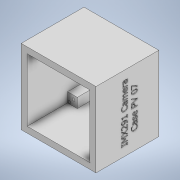
# Autodesk Inventor part: IMX291 Ethernet Strain Relief
Saved by Autodesk Inventor 2022.1 (Build 261234000, 234)
## iProperties
Created: 2021-07-23
Part Number: IMX291 Ethernet Strain Relief
Material: Generic
Document SubType Name: Modeling
Designer: robst
Density: 1 g/cm^3
Appearance: Default
Author: robst
Autodesk Inventor part; units mm, degrees
ref_plane "YZ Plane" through (0, 0, 0) normal (1, 0, 0) x (0, 1, 0)
ref_plane "XZ Plane" through (0, 0, 0) normal (0, 1, 0) x (-1, 0, 0)
ref_plane "XY Plane" through (0, 0, 0) normal (0, 0, 1) x (1, 0, 0)
sketch "Sketch8" plane through (0, 0, 0) normal (0, 0, 1) x (1, 0, 0)
  line L0 (-17, -17) -> (17, -17) construction
  line L1 (17, -17) -> (17, 17) construction
  line L2 (17, 17) -> (-17, 17) construction
  line L3 (-17, 17) -> (-17, -17) construction
  line L4 (-17, -17) -> (17, 17) construction
  line L5 (17, -17) -> (-17, 17) construction
  circle A0 centre (-17, 17) radius 0.889
  circle A1 centre (17, 17) radius 0.889
  circle A2 centre (17, -17) radius 0.889
  circle A3 centre (-17, -17) radius 0.889
  line L6 (-21, -21) -> (21, -21)
  line L7 (21, -21) -> (21, 21)
  line L8 (21, 21) -> (-21, 21)
  line L9 (-21, 21) -> (-21, -21)
  line L10 (-21, -21) -> (21, 21) construction
  line L11 (21, -21) -> (-21, 21) construction
  line L12 (-25, -25) -> (25, -25)
  line L13 (25, -25) -> (25, 25)
  line L14 (25, 25) -> (-25, 25)
  line L15 (-25, 25) -> (-25, -25)
  line L16 (-25, -25) -> (25, 25) construction
  line L17 (25, -25) -> (-25, 25) construction
  line L18 (0, 0) -> (9.8286, 0)
  line L19 (-14.5, -14.5) -> (14.5, -14.5) construction
  line L20 (14.5, -14.5) -> (14.5, 14.5) construction
  line L21 (14.5, 14.5) -> (-14.5, 14.5) construction
  line L22 (-14.5, 14.5) -> (-14.5, -14.5) construction
  line L23 (-14.5, -14.5) -> (14.5, 14.5) construction
  line L24 (14.5, -14.5) -> (-14.5, 14.5) construction
  line L25 (-21, 21) -> (-14.5, 21)
  line L26 (-14.5, 21) -> (-14.5, 14.5)
  line L27 (-14.5, 14.5) -> (-21, 14.5)
  line L28 (-21, 14.5) -> (-21, 21)
  line L29 (21, 21) -> (14.5, 21)
  line L30 (14.5, 21) -> (14.5, 14.5)
  line L31 (14.5, 14.5) -> (21, 14.5)
  line L32 (21, 14.5) -> (21, 21)
  line L33 (21, -21) -> (14.5, -21)
  line L34 (14.5, -21) -> (14.5, -14.5)
  line L35 (14.5, -14.5) -> (21, -14.5)
  line L36 (21, -14.5) -> (21, -21)
  line L37 (-21, -21) -> (-14.5, -21)
  line L38 (-14.5, -21) -> (-14.5, -14.5)
  line L39 (-14.5, -14.5) -> (-21, -14.5)
  line L40 (-21, -14.5) -> (-21, -21)
  point P0 (-25, 0)
  point P1 (-14.5, -21)
  dimension "d46" = 34
  dimension "d47" = 34
  dimension "d48" = 1.778
  dimension "d49" = 42
  dimension "d50" = 42
  dimension "d51" = 4
  dimension "d52" = 4
  dimension "d53" = 29
  dimension "d54" = 29
  dimension "d61" = 50
  dimension "d62" = 50
  constraints: 82 end point, 16 parallel, 9 midpoint, 8 horizontal, 8 perpendicular, 4 centre point, 4 coincident, 3 equal radius, 2 point on line
  measures "d46" distance of L0.start L0.end
  measures "d47" distance of L2.end L0.start
  measures "d48" diameter of A0
  measures "d49" distance of L7.end L8.end
  measures "d50" distance of L6.end L7.end
  measures "d51" distance between parallel lines of L8 L14
  measures "d52" distance from line of point (-25, 0) L9
  measures "d53" distance of L19.start L19.end
  measures "d54" distance of L20.end L19.end
  measures "d61" distance between parallel lines of L14 L12
  measures "d62" distance between parallel lines of L15 L13
extrude "Extrusion9" add sketch "Sketch8" against normal blind 15 contours L9 L39 L38 L6 | L34 L35 L7 L6 | L9 L8 L26 L27 | L31 L30 L8 L7 | L15 L14 L13 L12
sketch "Sketch9" plane through (0, 0, 0) normal (0, 0, 1) x (1, 0, 0)
  line L0 (21, 14.5) -> (21, -14.5) projected
  line L1 (-14.5, 21) -> (14.5, 21) projected
  line L2 (-21, -14.5) -> (-21, 14.5) projected
  line L3 (14.5, -21) -> (-14.5, -21) projected
  line L4 (-25, -25) -> (25, -25) projected
  line L5 (25, -25) -> (25, 25) projected
  line L6 (25, 25) -> (-25, 25) projected
  line L7 (-25, 25) -> (-25, -25) projected
  line L8 (-21, -21) -> (21, -21)
  line L9 (21, -21) -> (21, 21)
  line L10 (21, 21) -> (-21, 21)
  line L11 (-21, 21) -> (-21, -21)
  line L12 (-21, -21) -> (21, 21) construction
  line L13 (21, -21) -> (-21, 21) construction
  line L14 (-23, -23) -> (23, -23)
  line L15 (23, -23) -> (23, 23)
  line L16 (23, 23) -> (-23, 23)
  line L17 (-23, 23) -> (-23, -23)
  line L18 (-23, -23) -> (23, 23) construction
  line L19 (23, -23) -> (-23, 23) construction
  point P0 (0, 0)
  point P1 (-14.5, -21)
  constraints: 24 end point, 4 midpoint, 4 parallel, 2 perpendicular
extrude "Extrusion10" add sketch "Sketch9" along normal blind 27 contours L7 L6 L5 L4 | L17 L16 L15 L14
sketch "Sketch10" plane through (25, -25, -15) normal (1, 0, 0) x (0, 0, -1)
  line L0 (-42, 0) -> (0, 0) construction
  line L1 (-21, 0) -> (-21, 50) construction
  line L2 (0, 50) -> (-42, 50) construction
  line L3 (-21, 7.4068) -> (-21, 5.8574)
  line L4 (-21, 5.8574) -> (-21.4084, 5.8574)
  line L5 (-21.4084, 5.8574) -> (-21.4084, 6.3663)
  line L6 (-21.4084, 6.3663) -> (-24.5916, 6.3663)
  line L7 (-24.5916, 6.3663) -> (-24.5916, 5.8574)
  line L8 (-24.5916, 5.8574) -> (-25, 5.8574)
  line L9 (-25, 5.8574) -> (-25, 7.4068)
  line L10 (-25, 7.4068) -> (-24.5916, 7.4068)
  line L11 (-24.5916, 7.4068) -> (-24.5916, 6.8979)
  line L12 (-24.5916, 6.8979) -> (-21.4084, 6.8979)
  line L13 (-21.4084, 6.8979) -> (-21.4084, 7.4068)
  line L14 (-21.4084, 7.4068) -> (-21, 7.4068)
  line L15 (-21, 11.4943) -> (-21, 10.9627)
  line L16 (-21, 10.9627) -> (-24.4457, 10.9627)
  line L17 (-24.4457, 10.9627) -> (-22.1021, 9.919)
  line L18 (-22.1021, 9.919) -> (-22.1021, 9.5948)
  line L19 (-22.1021, 9.5948) -> (-24.4457, 8.5608)
  line L20 (-24.4457, 8.5608) -> (-21, 8.5608)
  line L21 (-21, 8.5608) -> (-21, 8.0648)
  line L22 (-21, 8.0648) -> (-25, 8.0648)
  line L23 (-25, 8.0648) -> (-25, 8.7909)
  line L24 (-25, 8.7909) -> (-22.7731, 9.7893)
  line L25 (-22.7731, 9.7893) -> (-25, 10.7553)
  line L26 (-25, 10.7553) -> (-25, 11.4943)
  line L27 (-25, 11.4943) -> (-21, 11.4943)
  line L28 (-21, 15.0697) -> (-21, 14.4603)
  line L29 (-21, 14.4603) -> (-22.5948, 13.4878)
  line L30 (-22.5948, 13.4878) -> (-21, 12.4959)
  line L31 (-21, 12.4959) -> (-21, 11.9222)
  line L32 (-21, 11.9222) -> (-23.0032, 13.1961)
  line L33 (-23.0032, 13.1961) -> (-25, 11.9611)
  line L34 (-25, 11.9611) -> (-25, 12.5705)
  line L35 (-25, 12.5705) -> (-23.4344, 13.5235)
  line L36 (-23.4344, 13.5235) -> (-25, 14.4959)
  line L37 (-25, 14.4959) -> (-25, 15.0697)
  line L38 (-25, 15.0697) -> (-23.0292, 13.8185)
  line L39 (-23.0292, 13.8185) -> (-21, 15.0697)
  line L40 (-21, 17.8509) -> (-21, 15.3841)
  line L41 (-21, 15.3841) -> (-21.5673, 15.3841)
  spline S0 degree 2 poles (-21.5673, 15.3841) (-21.8169, 15.6499) (-22.2804, 16.1232) (-22.53, 16.3501) knots 0 0 0 1 2 2 2
  spline S1 degree 2 poles (-22.53, 16.3501) (-23.0324, 16.8071) (-23.6353, 17.141) (-23.9562, 17.141) knots 0 0 0 1 2 2 2
  spline S2 degree 2 poles (-23.9562, 17.141) (-24.1248, 17.141) (-24.3776, 17.0373) (-24.4587, 16.9433) knots 0 0 0 1 2 2 2
  spline S3 degree 2 poles (-24.4587, 16.9433) (-24.5397, 16.8493) (-24.6207, 16.6029) (-24.6207, 16.4538) knots 0 0 0 1 2 2 2
  spline S4 degree 2 poles (-24.6207, 16.4538) (-24.6207, 16.3112) (-24.5494, 16.0194) (-24.4943, 15.8865) knots 0 0 0 1 2 2 2
  spline S5 degree 2 poles (-24.4943, 15.8865) (-24.4489, 15.7731) (-24.3193, 15.5624) (-24.2739, 15.4976) knots 0 0 0 1 2 2 2
  line L42 (-24.2739, 15.4976) -> (-24.2739, 15.4684)
  line L43 (-24.2739, 15.4684) -> (-24.8444, 15.4684)
  spline S6 degree 2 poles (-24.8444, 15.4684) (-24.9254, 15.6337) (-25.0843, 16.2269) (-25.0843, 16.4927) knots 0 0 0 1 2 2 2
  spline S7 degree 2 poles (-25.0843, 16.4927) (-25.0843, 17.0535) (-24.4911, 17.6856) (-23.9854, 17.6856) knots 0 0 0 1 2 2 2
  spline S8 degree 2 poles (-23.9854, 17.6856) (-23.7488, 17.6856) (-23.3533, 17.5754) (-23.1848, 17.4781) knots 0 0 0 1 2 2 2
  spline S9 degree 2 poles (-23.1848, 17.4781) (-23.0097, 17.3809) (-22.6661, 17.0989) (-22.5008, 16.9433) knots 0 0 0 1 2 2 2
  spline S10 degree 2 poles (-22.5008, 16.9433) (-22.2253, 16.6904) (-21.6353, 16.0713) (-21.4635, 15.8865) knots 0 0 0 1 2 2 2
  line L44 (-21.4635, 15.8865) -> (-21.4635, 17.8509)
  line L45 (-21.4635, 17.8509) -> (-21, 17.8509)
  spline S11 degree 2 poles (-23.7002, 18.2755) (-24.0081, 18.2755) (-24.5203, 18.4765) (-24.705, 18.6515) knots 0 0 0 1 2 2 2
  spline S12 degree 2 poles (-24.705, 18.6515) (-24.8833, 18.8169) (-25.081, 19.2998) (-25.081, 19.5462) knots 0 0 0 1 2 2 2
  spline S13 degree 2 poles (-25.081, 19.5462) (-25.081, 19.8217) (-24.8963, 20.269) (-24.7212, 20.4344) knots 0 0 0 1 2 2 2
  spline S14 degree 2 poles (-24.7212, 20.4344) (-24.5008, 20.6418) (-23.7877, 20.8687) (-23.2399, 20.8687) knots 0 0 0 1 2 2 2
  spline S15 degree 2 poles (-23.2399, 20.8687) (-22.7439, 20.8687) (-21.8558, 20.6451) (-21.5608, 20.4279) knots 0 0 0 1 2 2 2
  spline S16 degree 2 poles (-21.5608, 20.4279) (-21.2496, 20.1977) (-20.9222, 19.5494) (-20.9222, 19.0762) knots 0 0 0 1 2 2 2
  spline S17 degree 2 poles (-20.9222, 19.0762) (-20.9222, 18.9692) (-20.9449, 18.7261) (-20.9773, 18.6224) knots 0 0 0 1 2 2 2
  line L46 (-20.9773, 18.6224) -> (-21.4927, 18.6224)
  line L47 (-21.4927, 18.6224) -> (-21.4927, 18.6483)
  spline S18 degree 2 poles (-21.4927, 18.6483) (-21.4538, 18.7164) (-21.3857, 19.0016) (-21.3857, 19.1475) knots 0 0 0 1 2 2 2
  spline S19 degree 2 poles (-21.3857, 19.1475) (-21.3857, 19.6726) (-22.0794, 20.2723) (-22.7212, 20.3144) knots 0 0 0 1 2 2 2
  spline S20 degree 2 poles (-22.7212, 20.3144) (-22.5754, 20.1005) (-22.4425, 19.7115) (-22.4425, 19.4814) knots 0 0 0 1 2 2 2
  spline S21 degree 2 poles (-22.4425, 19.4814) (-22.4425, 19.2609) (-22.5397, 18.8947) (-22.6791, 18.7099) knots 0 0 0 1 2 2 2
  spline S22 degree 2 poles (-22.6791, 18.7099) (-22.8444, 18.4959) (-23.3468, 18.2755) (-23.7002, 18.2755) knots 0 0 0 1 2 2 2
  spline S23 degree 2 poles (-23.3598, 20.3274) (-23.765, 20.3274) (-24.2771, 20.1783) (-24.4165, 20.0454) knots 0 0 0 1 2 2 2
  spline S24 degree 2 poles (-24.4165, 20.0454) (-24.5462, 19.9287) (-24.6434, 19.6856) (-24.6434, 19.5429) knots 0 0 0 1 2 2 2
  spline S25 degree 2 poles (-24.6434, 19.5429) (-24.6434, 19.2123) (-24.1702, 18.8201) (-23.7229, 18.8201) knots 0 0 0 1 2 2 2
  spline S26 degree 2 poles (-23.7229, 18.8201) (-23.47, 18.8201) (-23.1426, 18.9498) (-23.0259, 19.0924) knots 0 0 0 1 2 2 2
  spline S27 degree 2 poles (-23.0259, 19.0924) (-22.9417, 19.1961) (-22.8865, 19.4522) (-22.8865, 19.6013) knots 0 0 0 1 2 2 2
  spline S28 degree 2 poles (-22.8865, 19.6013) (-22.8865, 19.7731) (-23.0065, 20.1686) (-23.107, 20.3177) knots 0 0 0 1 2 2 2
  spline S29 degree 2 poles (-23.107, 20.3177) (-23.1459, 20.3209) (-23.2788, 20.3274) (-23.3598, 20.3274) knots 0 0 0 1 2 2 2
  line L48 (-21, 23.6532) -> (-21, 21.7018)
  line L49 (-21, 21.7018) -> (-21.4084, 21.7018)
  line L50 (-21.4084, 21.7018) -> (-21.4084, 22.4279)
  line L51 (-21.4084, 22.4279) -> (-24.0891, 22.4279)
  line L52 (-24.0891, 22.4279) -> (-24.0891, 21.7018)
  line L53 (-24.0891, 21.7018) -> (-24.4554, 21.7018)
  spline S30 degree 2 poles (-24.4554, 21.7018) (-24.4554, 22.1135) (-24.6888, 22.5024) (-25.013, 22.5284) knots 0 0 0 1 2 2 2
  line L54 (-25.013, 22.5284) -> (-25.013, 22.9433)
  line L55 (-25.013, 22.9433) -> (-21.4084, 22.9433)
  line L56 (-21.4084, 22.9433) -> (-21.4084, 23.6532)
  line L57 (-21.4084, 23.6532) -> (-21, 23.6532)
  spline S31 degree 2 poles (-20.9287, 27.7828) (-20.9287, 27.3938) (-21.1912, 26.7358) (-21.4538, 26.4959) knots 0 0 0 1 2 2 2
  spline S32 degree 2 poles (-21.4538, 26.4959) (-21.7131, 26.2561) (-22.4911, 25.9935) (-22.9968, 25.9935) knots 0 0 0 1 2 2 2
  spline S33 degree 2 poles (-22.9968, 25.9935) (-23.4992, 25.9935) (-24.2447, 26.2496) (-24.5203, 26.4927) knots 0 0 0 1 2 2 2
  spline S34 degree 2 poles (-24.5203, 26.4927) (-24.7893, 26.7326) (-25.0713, 27.3874) (-25.0713, 27.7925) knots 0 0 0 1 2 2 2
  spline S35 degree 2 poles (-25.0713, 27.7925) (-25.0713, 27.9935) (-25.013, 28.3468) (-24.9676, 28.4959) knots 0 0 0 1 2 2 2
  spline S36 degree 2 poles (-24.9676, 28.4959) (-24.9254, 28.6256) (-24.8055, 28.8947) (-24.7342, 29.0276) knots 0 0 0 1 2 2 2
  line L58 (-24.7342, 29.0276) -> (-24.0924, 29.0276)
  line L59 (-24.0924, 29.0276) -> (-24.0924, 28.9854)
  spline S37 degree 2 poles (-24.0924, 28.9854) (-24.1572, 28.9141) (-24.3387, 28.6937) (-24.4263, 28.5348) knots 0 0 0 1 2 2 2
  spline S38 degree 2 poles (-24.4263, 28.5348) (-24.5105, 28.3825) (-24.6175, 28.0227) (-24.6175, 27.7893) knots 0 0 0 1 2 2 2
  spline S39 degree 2 poles (-24.6175, 27.7893) (-24.6175, 27.5332) (-24.4068, 27.0762) (-24.2058, 26.9044) knots 0 0 0 1 2 2 2
  spline S40 degree 2 poles (-24.2058, 26.9044) (-24.0016, 26.7358) (-23.3825, 26.5478) (-22.9968, 26.5478) knots 0 0 0 1 2 2 2
  spline S41 degree 2 poles (-22.9968, 26.5478) (-22.5851, 26.5478) (-21.9919, 26.7455) (-21.7877, 26.9173) knots 0 0 0 1 2 2 2
  spline S42 degree 2 poles (-21.7877, 26.9173) (-21.59, 27.0859) (-21.389, 27.5365) (-21.389, 27.7893) knots 0 0 0 1 2 2 2
  spline S43 degree 2 poles (-21.389, 27.7893) (-21.389, 28.0194) (-21.5024, 28.4117) (-21.5867, 28.564) knots 0 0 0 1 2 2 2
  spline S44 degree 2 poles (-21.5867, 28.564) (-21.671, 28.7099) (-21.846, 28.9271) (-21.9076, 28.9887) knots 0 0 0 1 2 2 2
  line L60 (-21.9076, 28.9887) -> (-21.9076, 29.0276)
  line L61 (-21.9076, 29.0276) -> (-21.2723, 29.0276)
  spline S45 degree 2 poles (-21.2723, 29.0276) (-21.2107, 28.8947) (-21.0972, 28.6613) (-21.0454, 28.4959) knots 0 0 0 1 2 2 2
  spline S46 degree 2 poles (-21.0454, 28.4959) (-20.987, 28.3209) (-20.9287, 28.0227) (-20.9287, 27.7828) knots 0 0 0 1 2 2 2
  spline S47 degree 2 poles (-21.3177, 31.1572) (-21.2723, 31.0956) (-21.1102, 30.8882) (-21.0616, 30.7909) knots 0 0 0 1 2 2 2
  spline S48 degree 2 poles (-21.0616, 30.7909) (-20.9903, 30.658) (-20.9157, 30.4084) (-20.9157, 30.1815) knots 0 0 0 1 2 2 2
  spline S49 degree 2 poles (-20.9157, 30.1815) (-20.9157, 29.9968) (-21.0551, 29.6629) (-21.1815, 29.5365) knots 0 0 0 1 2 2 2
  spline S50 degree 2 poles (-21.1815, 29.5365) (-21.3047, 29.4165) (-21.6677, 29.2707) (-21.8687, 29.2707) knots 0 0 0 1 2 2 2
  spline S51 degree 2 poles (-21.8687, 29.2707) (-22.1799, 29.2707) (-22.6207, 29.5332) (-22.7472, 29.8185) knots 0 0 0 1 2 2 2
  spline S52 degree 2 poles (-22.7472, 29.8185) (-22.8639, 30.0713) (-22.9514, 30.7585) (-22.9741, 31.1572) knots 0 0 0 1 2 2 2
  line L62 (-22.9741, 31.1572) -> (-23.0713, 31.1572)
  spline S53 degree 2 poles (-23.0713, 31.1572) (-23.2464, 31.1572) (-23.4635, 31.0502) (-23.5251, 30.953) knots 0 0 0 1 2 2 2
  spline S54 degree 2 poles (-23.5251, 30.953) (-23.5867, 30.8558) (-23.6256, 30.577) (-23.6256, 30.4279) knots 0 0 0 1 2 2 2
  spline S55 degree 2 poles (-23.6256, 30.4279) (-23.6256, 30.2528) (-23.5219, 29.7796) (-23.4214, 29.543) knots 0 0 0 1 2 2 2
  line L63 (-23.4214, 29.543) -> (-23.4214, 29.5138)
  line L64 (-23.4214, 29.5138) -> (-23.9368, 29.5138)
  spline S56 degree 2 poles (-23.9368, 29.5138) (-23.9757, 29.6532) (-24.0729, 30.175) (-24.0729, 30.4311) knots 0 0 0 1 2 2 2
  spline S57 degree 2 poles (-24.0729, 30.4311) (-24.0729, 30.7423) (-23.9757, 31.1669) (-23.8493, 31.3355) knots 0 0 0 1 2 2 2
  spline S58 degree 2 poles (-23.8493, 31.3355) (-23.7261, 31.5008) (-23.3339, 31.6629) (-23.0519, 31.6629) knots 0 0 0 1 2 2 2
  line L65 (-23.0519, 31.6629) -> (-21, 31.6629)
  line L66 (-21, 31.6629) -> (-21, 31.1572)
  line L67 (-21, 31.1572) -> (-21.3177, 31.1572)
  line L68 (-21.7391, 31.1572) -> (-22.5721, 31.1572)
  spline S59 degree 2 poles (-22.5721, 31.1572) (-22.5559, 30.9757) (-22.5008, 30.4279) (-22.4489, 30.2561) knots 0 0 0 1 2 2 2
  spline S60 degree 2 poles (-22.4489, 30.2561) (-22.3874, 30.0551) (-22.1313, 29.7925) (-21.9044, 29.7925) knots 0 0 0 1 2 2 2
  spline S61 degree 2 poles (-21.9044, 29.7925) (-21.6451, 29.7925) (-21.3825, 30.0843) (-21.3825, 30.363) knots 0 0 0 1 2 2 2
  spline S62 degree 2 poles (-21.3825, 30.363) (-21.3825, 30.5997) (-21.5867, 30.9887) (-21.7391, 31.1572) knots 0 0 0 1 2 2 2
  line L69 (-21, 35.7763) -> (-22.7374, 35.7763)
  spline S63 degree 2 poles (-22.7374, 35.7763) (-22.9449, 35.7763) (-23.2982, 35.7439) (-23.3955, 35.6921) knots 0 0 0 1 2 2 2
  spline S64 degree 2 poles (-23.3955, 35.6921) (-23.5024, 35.6402) (-23.6062, 35.4425) (-23.6062, 35.2707) knots 0 0 0 1 2 2 2
  spline S65 degree 2 poles (-23.6062, 35.2707) (-23.6062, 35.1151) (-23.4149, 34.7585) (-23.2334, 34.5705) knots 0 0 0 1 2 2 2
  spline S66 degree 2 poles (-23.2334, 34.5705) (-23.188, 34.5737) (-23.0616, 34.5802) (-22.9773, 34.5802) knots 0 0 0 1 2 2 2
  line L70 (-22.9773, 34.5802) -> (-21, 34.5802)
  line L71 (-21, 34.5802) -> (-21, 34.0746)
  line L72 (-21, 34.0746) -> (-22.7374, 34.0746)
  spline S67 degree 2 poles (-22.7374, 34.0746) (-22.9449, 34.0746) (-23.2982, 34.0421) (-23.3955, 33.9903) knots 0 0 0 1 2 2 2
  spline S68 degree 2 poles (-23.3955, 33.9903) (-23.5024, 33.9384) (-23.6062, 33.7407) (-23.6062, 33.5689) knots 0 0 0 1 2 2 2
  spline S69 degree 2 poles (-23.6062, 33.5689) (-23.6062, 33.4068) (-23.4019, 33.047) (-23.2431, 32.8784) knots 0 0 0 1 2 2 2
  line L73 (-23.2431, 32.8784) -> (-21, 32.8784)
  line L74 (-21, 32.8784) -> (-21, 32.3728)
  line L75 (-21, 32.3728) -> (-24.0016, 32.3728)
  line L76 (-24.0016, 32.3728) -> (-24.0016, 32.8784)
  line L77 (-24.0016, 32.8784) -> (-23.671, 32.8784)
  spline S70 degree 2 poles (-23.671, 32.8784) (-23.8687, 33.0762) (-24.0859, 33.4652) (-24.0859, 33.6985) knots 0 0 0 1 2 2 2
  spline S71 degree 2 poles (-24.0859, 33.6985) (-24.0859, 33.9643) (-23.8428, 34.376) (-23.5673, 34.483) knots 0 0 0 1 2 2 2
  spline S72 degree 2 poles (-23.5673, 34.483) (-23.8233, 34.7131) (-24.0859, 35.1475) (-24.0859, 35.4003) knots 0 0 0 1 2 2 2
  spline S73 degree 2 poles (-24.0859, 35.4003) (-24.0859, 35.5948) (-23.966, 35.9125) (-23.8298, 36.0292) knots 0 0 0 1 2 2 2
  spline S74 degree 2 poles (-23.8298, 36.0292) (-23.6937, 36.1491) (-23.2853, 36.282) (-22.9773, 36.282) knots 0 0 0 1 2 2 2
  line L78 (-22.9773, 36.282) -> (-21, 36.282)
  line L79 (-21, 36.282) -> (-21, 35.7763)
  spline S75 degree 2 poles (-20.9319, 38.295) (-20.9319, 37.5754) (-21.7391, 36.7844) (-22.4846, 36.7844) knots 0 0 0 1 2 2 2
  spline S76 degree 2 poles (-22.4846, 36.7844) (-23.2172, 36.7844) (-24.0859, 37.5527) (-24.0859, 38.1718) knots 0 0 0 1 2 2 2
  spline S77 degree 2 poles (-24.0859, 38.1718) (-24.0859, 38.4506) (-23.9238, 38.8817) (-23.752, 39.0405) knots 0 0 0 1 2 2 2
  spline S78 degree 2 poles (-23.752, 39.0405) (-23.5802, 39.2026) (-23.0843, 39.3744) (-22.7245, 39.3744) knots 0 0 0 1 2 2 2
  line L80 (-22.7245, 39.3744) -> (-22.4489, 39.3744)
  line L81 (-22.4489, 39.3744) -> (-22.4489, 37.2966)
  spline S79 degree 2 poles (-22.4489, 37.2966) (-21.9271, 37.2966) (-21.3728, 37.8217) (-21.3728, 38.2885) knots 0 0 0 1 2 2 2
  spline S80 degree 2 poles (-21.3728, 38.2885) (-21.3728, 38.4538) (-21.4473, 38.7747) (-21.5057, 38.9044) knots 0 0 0 1 2 2 2
  spline S81 degree 2 poles (-21.5057, 38.9044) (-21.5705, 39.0405) (-21.684, 39.2285) (-21.7358, 39.2901) knots 0 0 0 1 2 2 2
  line L82 (-21.7358, 39.2901) -> (-21.7358, 39.3193)
  line L83 (-21.7358, 39.3193) -> (-21.1848, 39.3193)
  spline S82 degree 2 poles (-21.1848, 39.3193) (-21.1491, 39.2318) (-21.0454, 38.966) (-21.0162, 38.8622) knots 0 0 0 1 2 2 2
  spline S83 degree 2 poles (-21.0162, 38.8622) (-20.9741, 38.7164) (-20.9319, 38.4765) (-20.9319, 38.295) knots 0 0 0 1 2 2 2
  spline S84 degree 2 poles (-22.8347, 38.8817) (-23.0389, 38.8752) (-23.3371, 38.7909) (-23.4376, 38.7099) knots 0 0 0 1 2 2 2
  spline S85 degree 2 poles (-23.4376, 38.7099) (-23.5511, 38.6224) (-23.671, 38.3468) (-23.671, 38.1426) knots 0 0 0 1 2 2 2
  spline S86 degree 2 poles (-23.671, 38.1426) (-23.671, 37.9417) (-23.5511, 37.6596) (-23.4344, 37.543) knots 0 0 0 1 2 2 2
  spline S87 degree 2 poles (-23.4344, 37.543) (-23.3144, 37.4295) (-23.0259, 37.3128) (-22.8347, 37.2966) knots 0 0 0 1 2 2 2
  line L84 (-22.8347, 37.2966) -> (-22.8347, 38.8817)
  line L85 (-23.4603, 41.4781) -> (-23.4603, 41.4522)
  spline S88 degree 2 poles (-23.4603, 41.4522) (-23.4765, 41.3938) (-23.483, 41.2674) (-23.483, 41.1799) knots 0 0 0 1 2 2 2
  spline S89 degree 2 poles (-23.483, 41.1799) (-23.483, 40.9757) (-23.3047, 40.5737) (-23.1297, 40.3922) knots 0 0 0 1 2 2 2
  line L86 (-23.1297, 40.3922) -> (-21, 40.3922)
  line L87 (-21, 40.3922) -> (-21, 39.8865)
  line L88 (-21, 39.8865) -> (-24.0016, 39.8865)
  line L89 (-24.0016, 39.8865) -> (-24.0016, 40.3922)
  line L90 (-24.0016, 40.3922) -> (-23.5543, 40.3922)
  spline S90 degree 2 poles (-23.5543, 40.3922) (-23.8006, 40.6677) (-24.0016, 41.0794) (-24.0016, 41.2739) knots 0 0 0 1 2 2 2
  spline S91 degree 2 poles (-24.0016, 41.2739) (-24.0016, 41.3517) (-23.9951, 41.4295) (-23.9854, 41.4781) knots 0 0 0 1 2 2 2
  line L91 (-23.9854, 41.4781) -> (-23.4603, 41.4781)
  spline S92 degree 2 poles (-21.3177, 43.543) (-21.2723, 43.4814) (-21.1102, 43.2739) (-21.0616, 43.1767) knots 0 0 0 1 2 2 2
  spline S93 degree 2 poles (-21.0616, 43.1767) (-20.9903, 43.0438) (-20.9157, 42.7942) (-20.9157, 42.5673) knots 0 0 0 1 2 2 2
  spline S94 degree 2 poles (-20.9157, 42.5673) (-20.9157, 42.3825) (-21.0551, 42.0486) (-21.1815, 41.9222) knots 0 0 0 1 2 2 2
  spline S95 degree 2 poles (-21.1815, 41.9222) (-21.3047, 41.8023) (-21.6677, 41.6564) (-21.8687, 41.6564) knots 0 0 0 1 2 2 2
  spline S96 degree 2 poles (-21.8687, 41.6564) (-22.1799, 41.6564) (-22.6207, 41.919) (-22.7472, 42.2042) knots 0 0 0 1 2 2 2
  spline S97 degree 2 poles (-22.7472, 42.2042) (-22.8639, 42.4571) (-22.9514, 43.1442) (-22.9741, 43.543) knots 0 0 0 1 2 2 2
  line L92 (-22.9741, 43.543) -> (-23.0713, 43.543)
  spline S98 degree 2 poles (-23.0713, 43.543) (-23.2464, 43.543) (-23.4635, 43.436) (-23.5251, 43.3387) knots 0 0 0 1 2 2 2
  spline S99 degree 2 poles (-23.5251, 43.3387) (-23.5867, 43.2415) (-23.6256, 42.9627) (-23.6256, 42.8136) knots 0 0 0 1 2 2 2
  spline S100 degree 2 poles (-23.6256, 42.8136) (-23.6256, 42.6386) (-23.5219, 42.1653) (-23.4214, 41.9287) knots 0 0 0 1 2 2 2
  line L93 (-23.4214, 41.9287) -> (-23.4214, 41.8995)
  line L94 (-23.4214, 41.8995) -> (-23.9368, 41.8995)
  spline S101 degree 2 poles (-23.9368, 41.8995) (-23.9757, 42.0389) (-24.0729, 42.5608) (-24.0729, 42.8169) knots 0 0 0 1 2 2 2
  spline S102 degree 2 poles (-24.0729, 42.8169) (-24.0729, 43.128) (-23.9757, 43.5527) (-23.8493, 43.7212) knots 0 0 0 1 2 2 2
  spline S103 degree 2 poles (-23.8493, 43.7212) (-23.7261, 43.8865) (-23.3339, 44.0486) (-23.0519, 44.0486) knots 0 0 0 1 2 2 2
  line L95 (-23.0519, 44.0486) -> (-21, 44.0486)
  line L96 (-21, 44.0486) -> (-21, 43.543)
  line L97 (-21, 43.543) -> (-21.3177, 43.543)
  line L98 (-21.7391, 43.543) -> (-22.5721, 43.543)
  spline S104 degree 2 poles (-22.5721, 43.543) (-22.5559, 43.3614) (-22.5008, 42.8136) (-22.4489, 42.6418) knots 0 0 0 1 2 2 2
  spline S105 degree 2 poles (-22.4489, 42.6418) (-22.3874, 42.4408) (-22.1313, 42.1783) (-21.9044, 42.1783) knots 0 0 0 1 2 2 2
  spline S106 degree 2 poles (-21.9044, 42.1783) (-21.6451, 42.1783) (-21.3825, 42.47) (-21.3825, 42.7488) knots 0 0 0 1 2 2 2
  spline S107 degree 2 poles (-21.3825, 42.7488) (-21.3825, 42.9854) (-21.5867, 43.3744) (-21.7391, 43.543) knots 0 0 0 1 2 2 2
  spline S108 degree 2 poles (-14.3265, 13.3193) (-14.3265, 12.9303) (-14.5891, 12.2723) (-14.8516, 12.0324) knots 0 0 0 1 2 2 2
  spline S109 degree 2 poles (-14.8516, 12.0324) (-15.1109, 11.7925) (-15.8889, 11.53) (-16.3946, 11.53) knots 0 0 0 1 2 2 2
  spline S110 degree 2 poles (-16.3946, 11.53) (-16.897, 11.53) (-17.6425, 11.7861) (-17.9181, 12.0292) knots 0 0 0 1 2 2 2
  spline S111 degree 2 poles (-17.9181, 12.0292) (-18.1871, 12.269) (-18.4691, 12.9238) (-18.4691, 13.329) knots 0 0 0 1 2 2 2
  spline S112 degree 2 poles (-18.4691, 13.329) (-18.4691, 13.53) (-18.4108, 13.8833) (-18.3654, 14.0324) knots 0 0 0 1 2 2 2
  spline S113 degree 2 poles (-18.3654, 14.0324) (-18.3233, 14.1621) (-18.2033, 14.4311) (-18.132, 14.564) knots 0 0 0 1 2 2 2
  line L99 (-18.132, 14.564) -> (-17.4902, 14.564)
  line L100 (-17.4902, 14.564) -> (-17.4902, 14.5219)
  spline S114 degree 2 poles (-17.4902, 14.5219) (-17.555, 14.4506) (-17.7365, 14.2301) (-17.8241, 14.0713) knots 0 0 0 1 2 2 2
  spline S115 degree 2 poles (-17.8241, 14.0713) (-17.9083, 13.919) (-18.0153, 13.5592) (-18.0153, 13.3258) knots 0 0 0 1 2 2 2
  spline S116 degree 2 poles (-18.0153, 13.3258) (-18.0153, 13.0697) (-17.8046, 12.6126) (-17.6036, 12.4408) knots 0 0 0 1 2 2 2
  spline S117 degree 2 poles (-17.6036, 12.4408) (-17.3994, 12.2723) (-16.7803, 12.0843) (-16.3946, 12.0843) knots 0 0 0 1 2 2 2
  spline S118 degree 2 poles (-16.3946, 12.0843) (-15.9829, 12.0843) (-15.3897, 12.282) (-15.1855, 12.4538) knots 0 0 0 1 2 2 2
  spline S119 degree 2 poles (-15.1855, 12.4538) (-14.9878, 12.6224) (-14.7868, 13.0729) (-14.7868, 13.3258) knots 0 0 0 1 2 2 2
  spline S120 degree 2 poles (-14.7868, 13.3258) (-14.7868, 13.5559) (-14.9002, 13.9481) (-14.9845, 14.1005) knots 0 0 0 1 2 2 2
  spline S121 degree 2 poles (-14.9845, 14.1005) (-15.0688, 14.2464) (-15.2438, 14.4635) (-15.3054, 14.5251) knots 0 0 0 1 2 2 2
  line L101 (-15.3054, 14.5251) -> (-15.3054, 14.564)
  line L102 (-15.3054, 14.564) -> (-14.6701, 14.564)
  spline S122 degree 2 poles (-14.6701, 14.564) (-14.6085, 14.4311) (-14.495, 14.1977) (-14.4432, 14.0324) knots 0 0 0 1 2 2 2
  spline S123 degree 2 poles (-14.4432, 14.0324) (-14.3848, 13.8574) (-14.3265, 13.5592) (-14.3265, 13.3193) knots 0 0 0 1 2 2 2
  spline S124 degree 2 poles (-14.7155, 16.6937) (-14.6701, 16.6321) (-14.508, 16.4246) (-14.4594, 16.3274) knots 0 0 0 1 2 2 2
  spline S125 degree 2 poles (-14.4594, 16.3274) (-14.3881, 16.1945) (-14.3135, 15.9449) (-14.3135, 15.718) knots 0 0 0 1 2 2 2
  spline S126 degree 2 poles (-14.3135, 15.718) (-14.3135, 15.5332) (-14.4529, 15.1994) (-14.5793, 15.0729) knots 0 0 0 1 2 2 2
  spline S127 degree 2 poles (-14.5793, 15.0729) (-14.7025, 14.953) (-15.0656, 14.8071) (-15.2665, 14.8071) knots 0 0 0 1 2 2 2
  spline S128 degree 2 poles (-15.2665, 14.8071) (-15.5777, 14.8071) (-16.0186, 15.0697) (-16.145, 15.3549) knots 0 0 0 1 2 2 2
  spline S129 degree 2 poles (-16.145, 15.3549) (-16.2617, 15.6078) (-16.3492, 16.295) (-16.3719, 16.6937) knots 0 0 0 1 2 2 2
  line L103 (-16.3719, 16.6937) -> (-16.4691, 16.6937)
  spline S130 degree 2 poles (-16.4691, 16.6937) (-16.6442, 16.6937) (-16.8613, 16.5867) (-16.9229, 16.4895) knots 0 0 0 1 2 2 2
  spline S131 degree 2 poles (-16.9229, 16.4895) (-16.9845, 16.3922) (-17.0234, 16.1135) (-17.0234, 15.9643) knots 0 0 0 1 2 2 2
  spline S132 degree 2 poles (-17.0234, 15.9643) (-17.0234, 15.7893) (-16.9197, 15.316) (-16.8192, 15.0794) knots 0 0 0 1 2 2 2
  line L104 (-16.8192, 15.0794) -> (-16.8192, 15.0502)
  line L105 (-16.8192, 15.0502) -> (-17.3346, 15.0502)
  spline S133 degree 2 poles (-17.3346, 15.0502) (-17.3735, 15.1896) (-17.4707, 15.7115) (-17.4707, 15.9676) knots 0 0 0 1 2 2 2
  spline S134 degree 2 poles (-17.4707, 15.9676) (-17.4707, 16.2788) (-17.3735, 16.7034) (-17.2471, 16.872) knots 0 0 0 1 2 2 2
  spline S135 degree 2 poles (-17.2471, 16.872) (-17.1239, 17.0373) (-16.7317, 17.1994) (-16.4497, 17.1994) knots 0 0 0 1 2 2 2
  line L106 (-16.4497, 17.1994) -> (-14.3978, 17.1994)
  line L107 (-14.3978, 17.1994) -> (-14.3978, 16.6937)
  line L108 (-14.3978, 16.6937) -> (-14.7155, 16.6937)
  line L109 (-15.1369, 16.6937) -> (-15.9699, 16.6937)
  spline S136 degree 2 poles (-15.9699, 16.6937) (-15.9537, 16.5122) (-15.8986, 15.9643) (-15.8468, 15.7925) knots 0 0 0 1 2 2 2
  spline S137 degree 2 poles (-15.8468, 15.7925) (-15.7852, 15.5916) (-15.5291, 15.329) (-15.3022, 15.329) knots 0 0 0 1 2 2 2
  spline S138 degree 2 poles (-15.3022, 15.329) (-15.0429, 15.329) (-14.7803, 15.6207) (-14.7803, 15.8995) knots 0 0 0 1 2 2 2
  spline S139 degree 2 poles (-14.7803, 15.8995) (-14.7803, 16.1361) (-14.9845, 16.5251) (-15.1369, 16.6937) knots 0 0 0 1 2 2 2
  spline S140 degree 2 poles (-14.3265, 18.7196) (-14.3265, 18.4182) (-14.4886, 17.8963) (-14.5793, 17.7245) knots 0 0 0 1 2 2 2
  line L110 (-14.5793, 17.7245) -> (-15.1466, 17.7245)
  line L111 (-15.1466, 17.7245) -> (-15.1466, 17.7504)
  spline S141 degree 2 poles (-15.1466, 17.7504) (-15.0947, 17.8152) (-14.9715, 17.9903) (-14.9035, 18.1361) knots 0 0 0 1 2 2 2
  spline S142 degree 2 poles (-14.9035, 18.1361) (-14.8419, 18.2626) (-14.7511, 18.5737) (-14.7511, 18.7391) knots 0 0 0 1 2 2 2
  spline S143 degree 2 poles (-14.7511, 18.7391) (-14.7511, 18.859) (-14.8062, 19.1345) (-14.8516, 19.1994) knots 0 0 0 1 2 2 2
  spline S144 degree 2 poles (-14.8516, 19.1994) (-14.9132, 19.2934) (-15.0526, 19.3776) (-15.1952, 19.3776) knots 0 0 0 1 2 2 2
  spline S145 degree 2 poles (-15.1952, 19.3776) (-15.3735, 19.3776) (-15.5583, 19.1831) (-15.6198, 18.9335) knots 0 0 0 1 2 2 2
  spline S146 degree 2 poles (-15.6198, 18.9335) (-15.6425, 18.8363) (-15.7074, 18.5251) (-15.743, 18.3922) knots 0 0 0 1 2 2 2
  spline S147 degree 2 poles (-15.743, 18.3922) (-15.8435, 18.0486) (-16.2584, 17.7374) (-16.5534, 17.7374) knots 0 0 0 1 2 2 2
  spline S148 degree 2 poles (-16.5534, 17.7374) (-16.9618, 17.7374) (-17.4707, 18.3501) (-17.4707, 18.8558) knots 0 0 0 1 2 2 2
  spline S149 degree 2 poles (-17.4707, 18.8558) (-17.4707, 19.1053) (-17.3476, 19.611) (-17.2536, 19.7828) knots 0 0 0 1 2 2 2
  line L112 (-17.2536, 19.7828) -> (-16.7122, 19.7828)
  line L113 (-16.7122, 19.7828) -> (-16.7122, 19.7569)
  spline S150 degree 2 poles (-16.7122, 19.7569) (-16.8678, 19.5624) (-17.0461, 19.0891) (-17.0461, 18.846) knots 0 0 0 1 2 2 2
  spline S151 degree 2 poles (-17.0461, 18.846) (-17.0461, 18.5964) (-16.8354, 18.2528) (-16.6247, 18.2528) knots 0 0 0 1 2 2 2
  spline S152 degree 2 poles (-16.6247, 18.2528) (-16.4335, 18.2528) (-16.2487, 18.457) (-16.1903, 18.684) knots 0 0 0 1 2 2 2
  spline S153 degree 2 poles (-16.1903, 18.684) (-16.1612, 18.7942) (-16.1028, 19.0729) (-16.0672, 19.2253) knots 0 0 0 1 2 2 2
  spline S154 degree 2 poles (-16.0672, 19.2253) (-15.9829, 19.5559) (-15.5972, 19.893) (-15.2633, 19.893) knots 0 0 0 1 2 2 2
  spline S155 degree 2 poles (-15.2633, 19.893) (-15.0688, 19.893) (-14.7252, 19.7407) (-14.5988, 19.5916) knots 0 0 0 1 2 2 2
  spline S156 degree 2 poles (-14.5988, 19.5916) (-14.4659, 19.4327) (-14.3265, 19.0276) (-14.3265, 18.7196) knots 0 0 0 1 2 2 2
  spline S157 degree 2 poles (-14.3297, 21.6661) (-14.3297, 20.9465) (-15.1369, 20.1556) (-15.8824, 20.1556) knots 0 0 0 1 2 2 2
  spline S158 degree 2 poles (-15.8824, 20.1556) (-16.615, 20.1556) (-17.4837, 20.9238) (-17.4837, 21.5429) knots 0 0 0 1 2 2 2
  spline S159 degree 2 poles (-17.4837, 21.5429) (-17.4837, 21.8217) (-17.3216, 22.2528) (-17.1498, 22.4117) knots 0 0 0 1 2 2 2
  spline S160 degree 2 poles (-17.1498, 22.4117) (-16.978, 22.5737) (-16.4821, 22.7455) (-16.1223, 22.7455) knots 0 0 0 1 2 2 2
  line L114 (-16.1223, 22.7455) -> (-15.8468, 22.7455)
  line L115 (-15.8468, 22.7455) -> (-15.8468, 20.6677)
  spline S161 degree 2 poles (-15.8468, 20.6677) (-15.3249, 20.6677) (-14.7706, 21.1929) (-14.7706, 21.6596) knots 0 0 0 1 2 2 2
  spline S162 degree 2 poles (-14.7706, 21.6596) (-14.7706, 21.825) (-14.8451, 22.1459) (-14.9035, 22.2755) knots 0 0 0 1 2 2 2
  spline S163 degree 2 poles (-14.9035, 22.2755) (-14.9683, 22.4117) (-15.0818, 22.5997) (-15.1336, 22.6613) knots 0 0 0 1 2 2 2
  line L116 (-15.1336, 22.6613) -> (-15.1336, 22.6904)
  line L117 (-15.1336, 22.6904) -> (-14.5826, 22.6904)
  spline S164 degree 2 poles (-14.5826, 22.6904) (-14.5469, 22.6029) (-14.4432, 22.3371) (-14.414, 22.2334) knots 0 0 0 1 2 2 2
  spline S165 degree 2 poles (-14.414, 22.2334) (-14.3719, 22.0875) (-14.3297, 21.8476) (-14.3297, 21.6661) knots 0 0 0 1 2 2 2
  spline S166 degree 2 poles (-16.2325, 22.2528) (-16.4367, 22.2464) (-16.7349, 22.1621) (-16.8354, 22.081) knots 0 0 0 1 2 2 2
  spline S167 degree 2 poles (-16.8354, 22.081) (-16.9489, 21.9935) (-17.0688, 21.718) (-17.0688, 21.5138) knots 0 0 0 1 2 2 2
  spline S168 degree 2 poles (-17.0688, 21.5138) (-17.0688, 21.3128) (-16.9489, 21.0308) (-16.8322, 20.9141) knots 0 0 0 1 2 2 2
  spline S169 degree 2 poles (-16.8322, 20.9141) (-16.7122, 20.8006) (-16.4237, 20.684) (-16.2325, 20.6677) knots 0 0 0 1 2 2 2
  line L118 (-16.2325, 20.6677) -> (-16.2325, 22.2528)
  spline S170 degree 2 poles (-17.192, 27.5429) (-16.9327, 27.5429) (-16.4659, 27.3582) (-16.3038, 27.1929) knots 0 0 0 1 2 2 2
  spline S171 degree 2 poles (-16.3038, 27.1929) (-16.0996, 26.9854) (-15.8889, 26.4246) (-15.8889, 25.9968) knots 0 0 0 1 2 2 2
  line L119 (-15.8889, 25.9968) -> (-15.8889, 25.5462)
  line L120 (-15.8889, 25.5462) -> (-14.3978, 25.5462)
  line L121 (-14.3978, 25.5462) -> (-14.3978, 25.0146)
  line L122 (-14.3978, 25.0146) -> (-18.3978, 25.0146)
  line L123 (-18.3978, 25.0146) -> (-18.3978, 26.0194)
  spline S172 degree 2 poles (-18.3978, 26.0194) (-18.3978, 26.376) (-18.2811, 26.8752) (-18.1482, 27.0665) knots 0 0 0 1 2 2 2
  spline S173 degree 2 poles (-18.1482, 27.0665) (-17.9959, 27.2901) (-17.5258, 27.5429) (-17.192, 27.5429) knots 0 0 0 1 2 2 2
  spline S174 degree 2 poles (-17.1758, 26.9887) (-17.3832, 26.9887) (-17.6879, 26.846) (-17.7852, 26.7002) knots 0 0 0 1 2 2 2
  spline S175 degree 2 poles (-17.7852, 26.7002) (-17.8694, 26.5737) (-17.9375, 26.2366) (-17.9375, 25.987) knots 0 0 0 1 2 2 2
  line L124 (-17.9375, 25.987) -> (-17.9375, 25.5462)
  line L125 (-17.9375, 25.5462) -> (-16.3427, 25.5462)
  line L126 (-16.3427, 25.5462) -> (-16.3427, 25.9092)
  spline S176 degree 2 poles (-16.3427, 25.9092) (-16.3427, 26.2334) (-16.4464, 26.6321) (-16.5826, 26.7618) knots 0 0 0 1 2 2 2
  spline S177 degree 2 poles (-16.5826, 26.7618) (-16.7025, 26.8817) (-16.9845, 26.9887) (-17.1758, 26.9887) knots 0 0 0 1 2 2 2
  line L127 (-18.3978, 30.9498) -> (-14.3978, 29.5721)
  line L128 (-14.3978, 29.5721) -> (-14.3978, 28.9984)
  line L129 (-14.3978, 28.9984) -> (-18.3978, 27.6207)
  line L130 (-18.3978, 27.6207) -> (-18.3978, 28.1912)
  line L131 (-18.3978, 28.1912) -> (-15.0753, 29.2998)
  line L132 (-15.0753, 29.2998) -> (-18.3978, 30.4084)
  line L133 (-18.3978, 30.4084) -> (-18.3978, 30.9498)
  spline S178 degree 2 poles (-16.3978, 35.4716) (-15.3216, 35.4716) (-14.3135, 34.846) (-14.3135, 34.1945) knots 0 0 0 1 2 2 2
  spline S179 degree 2 poles (-14.3135, 34.1945) (-14.3135, 33.5332) (-15.3411, 32.9141) (-16.3946, 32.9141) knots 0 0 0 1 2 2 2
  spline S180 degree 2 poles (-16.3946, 32.9141) (-17.4772, 32.9141) (-18.4788, 33.5397) (-18.4788, 34.1945) knots 0 0 0 1 2 2 2
  spline S181 degree 2 poles (-18.4788, 34.1945) (-18.4788, 34.8525) (-17.4416, 35.4716) (-16.3978, 35.4716) knots 0 0 0 1 2 2 2
  spline S182 degree 2 poles (-15.179, 34.7844) (-15.3767, 34.8622) (-15.9861, 34.9271) (-16.3978, 34.9271) knots 0 0 0 1 2 2 2
  spline S183 degree 2 poles (-16.3978, 34.9271) (-16.8095, 34.9271) (-17.4156, 34.8622) (-17.6198, 34.7812) knots 0 0 0 1 2 2 2
  spline S184 degree 2 poles (-17.6198, 34.7812) (-17.8241, 34.7002) (-18.0348, 34.4182) (-18.0348, 34.1945) knots 0 0 0 1 2 2 2
  spline S185 degree 2 poles (-18.0348, 34.1945) (-18.0348, 33.9708) (-17.8241, 33.6823) (-17.6134, 33.5981) knots 0 0 0 1 2 2 2
  spline S186 degree 2 poles (-17.6134, 33.5981) (-17.4091, 33.517) (-16.7868, 33.4587) (-16.3946, 33.4587) knots 0 0 0 1 2 2 2
  spline S187 degree 2 poles (-16.3946, 33.4587) (-15.9732, 33.4587) (-15.4091, 33.5105) (-15.1887, 33.5948) knots 0 0 0 1 2 2 2
  spline S188 degree 2 poles (-15.1887, 33.5948) (-14.9813, 33.6726) (-14.7576, 33.9611) (-14.7576, 34.1945) knots 0 0 0 1 2 2 2
  spline S189 degree 2 poles (-14.7576, 34.1945) (-14.7576, 34.4149) (-14.9683, 34.7034) (-15.179, 34.7844) knots 0 0 0 1 2 2 2
  line L134 (-17.7981, 38.4959) -> (-14.3978, 36.765)
  line L135 (-14.3978, 36.765) -> (-14.3978, 36.1945)
  line L136 (-14.3978, 36.1945) -> (-17.9278, 38.0227)
  line L137 (-17.9278, 38.0227) -> (-17.9278, 35.9579)
  line L138 (-17.9278, 35.9579) -> (-18.3978, 35.9579)
  line L139 (-18.3978, 35.9579) -> (-18.3978, 38.4959)
  line L140 (-18.3978, 38.4959) -> (-17.7981, 38.4959)
  point P0 (-15, 25)
  constraints: 2 end point, 2 midpoint, 1 vertical
emboss "Emboss2" sketch "Sketch10" operation cut depth 1 direction (-1, 0, 0)
sketch "Sketch11" plane through (0, 0, -15) normal (0, 0, -1) x (-1, 0, 0)
  line L0 (25, -25) -> (25, 25) projected
  line L1 (-25, -25) -> (25, -25) projected
  line L2 (-25, 25) -> (-25, -25) projected
  line L3 (25, 25) -> (-25, 25) projected
  line L4 (-19.75, 19.75) -> (-19.75, -19.75) construction
  line L5 (-19.75, -19.75) -> (19.75, -19.75) construction
  line L6 (19.75, -19.75) -> (19.75, 19.75) construction
  line L7 (19.75, 19.75) -> (-19.75, 19.75) construction
  line L8 (-19.75, 19.75) -> (19.75, -19.75) construction
  line L9 (-19.75, -19.75) -> (19.75, 19.75) construction
  point P0 (0, 0)
  dimension "d74" = 39.5
  dimension "d75" = 39.5
  constraints: 12 end point, 4 coincident, 2 midpoint, 2 parallel, 1 perpendicular, 1 vertical
  measures "d74" distance of L5.end L6.end
  measures "d75" distance of L6.end L4.start
hole "Hole1" at (-19.75, 19.75, -15) at (-19.75, -19.75, -15) at (19.75, -19.75, -15) at (19.75, 19.75, -15) direction (0, 0, 1) diameter 1.6942 end through all thread size "2-56 UNC" class "2B" standard "ANSI Unified Screw Threads"
equation "\"d46\" = screwSpacing"
equation "\"d47\" = screwSpacing"
equation "\"d48\" = holeDiameter"
equation "\"d49\" = interiorWidth"
equation "\"d50\" = interiorWidth"
equation "\"d51\" = sideWallThickness"
equation "\"d52\" = sideWallThickness"
equation "\"screwSpacing\" = 34"
equation "\"interiorWidth\" = 42"
equation "\"bottomWallThickness\" = 2"
equation "\"holeDiameter\" = 1.778"
equation "\"sideWallThickness\" = 4"
body "Solid4"
body "Solid5"
